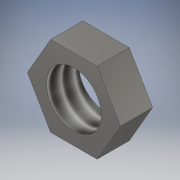
# Autodesk Inventor part: Nut
Saved by Autodesk Inventor 2018 (Build 220112000, 112)
## iProperties
Created: 2018-05-07
Part Number: Nut
Material: Stainless Steel
Document SubType Name: Modeling
Designer: 232963
Density: 8 g/cm^3
Appearance: Semi-Polished
Author: 232963
Autodesk Inventor part; units mm, degrees
ref_plane "YZ Plane" through (0, 0, 0) normal (1, 0, 0) x (0, 1, 0)
ref_plane "XZ Plane" through (0, 0, 0) normal (0, 1, 0) x (-1, 0, 0)
ref_plane "XY Plane" through (0, 0, 0) normal (0, 0, 1) x (1, 0, 0)
sketch "Sketch1" plane through (0, 0, 0) normal (0, 0, 1) x (1, 0, 0)
  line L0 (3.6662, 0) -> (1.8331, -3.175)
  line L1 (1.8331, -3.175) -> (-1.8331, -3.175)
  line L2 (-1.8331, -3.175) -> (-3.6662, 0)
  line L3 (-3.6662, 0) -> (-1.8331, 3.175)
  line L4 (-1.8331, 3.175) -> (1.8331, 3.175)
  line L5 (1.8331, 3.175) -> (3.6662, 0)
  circle A0 centre (0, 0) radius 2.159
  point P0 (0, 0)
  point P1 (0, 0)
  dimension "d0" = 6.35
  dimension "d1" = 4.318
  constraints: 12 end point, 1 centre point, 1 coincident, 13 other
  measures "d0" distance between parallel lines of L1 L4
  measures "d1" diameter of A0
extrude "Extrusion1" add sketch "Sketch1" along normal blind 2.54
thread "Thread1" size "10-24 UNC" class "2B" standard "ANSI Unified Screw Threads" full length
body "Solid1"
